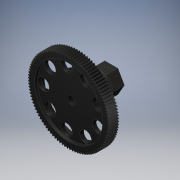
# Autodesk Inventor part: RoueDentée
Saved by Autodesk Inventor 2019 (Build 230136000, 136)
## iProperties
Created: 2019-07-30
Part Number: RoueDentée
Material: Plastique ABS
Document SubType Name: Modeling
Designer: Sébastien DI MERCURIO
Mass: 7.34284 g
Surface Area: 34.3062 cm^2
Volume: 6.92721 cm^3
Density: 1.06 g/cm^3
Appearance: Lustré - Noir
Author: Sébastien DI MERCURIO
Autodesk Inventor part; units mm, degrees
ref_plane "YZ Plane" through (0, 0, 0) normal (1, 0, 0) x (0, 1, 0)
ref_plane "XZ Plane" through (0, 0, 0) normal (0, 1, 0) x (-1, 0, 0)
ref_plane "XY Plane" through (0, 0, 0) normal (0, 0, 1) x (1, 0, 0)
sketch "Esquisse1" plane through (0, 0, 0) normal (0, 0, 1) x (1, 0, 0)
  circle A0 centre (0, 0) radius 21
  dimension "d0" = 42
  constraints: 1 centre point, 1 coincident
  measures "d0" diameter of A0
extrude "Extrusion1" add sketch "Esquisse1" along normal blind 5
sketch "Esquisse2" plane through (0, 0, 5) normal (0, 0, 1) x (1, 0, 0)
  circle A0 centre (0, 0) radius 17.5
  circle A1 centre (0, 0) radius 21 projected
  dimension "d3" = 3.5
  constraints: 1 centre point, 1 coincident
  measures "d3" radial gap between concentric circles of A0 A1
extrude "Extrusion2" cut sketch "Esquisse2" against normal blind 1.5 contours A0
sketch "Esquisse3" plane through (0, 0, 0) normal (0, 0, -1) x (-1, 0, 0)
  circle A0 centre (0, 0) radius 17.5
  circle A1 centre (0, 0) radius 21 projected
  dimension "d6" = 3.5
  constraints: 1 centre point, 1 coincident
  measures "d6" radial gap between concentric circles of A0 A1
extrude "Extrusion3" cut sketch "Esquisse3" against normal blind 1.5 contours A0
sketch "Esquisse4" plane through (0, 0, 1.5) normal (0, 0, -1) x (-1, 0, 0)
  circle A0 centre (0, 0) radius 14.5 construction
  circle A1 centre (14.5, 0) radius 3
  circle A2 centre (11.1076, 9.3204) radius 3
  circle A3 centre (2.5179, 14.2797) radius 3
  circle A4 centre (-7.25, 12.5574) radius 3
  circle A5 centre (-13.6255, 4.9593) radius 3
  circle A6 centre (-13.6255, -4.9593) radius 3
  circle A7 centre (-7.25, -12.5574) radius 3
  circle A8 centre (2.5179, -14.2797) radius 3
  circle A9 centre (11.1076, -9.3204) radius 3
  dimension "d9" = 29
  dimension "d10" = 6
  dimension "d13" = 360
  constraints: 9 centre point, 2 horizontal alignment, 1 coincident, 21 other
  measures "d10" diameter of A1
extrude "Extrusion4" cut sketch "Esquisse4" against normal through all
sketch "Esquisse5" plane through (0, 0, 1.5) normal (0, 0, -1) x (-1, 0, 0)
  circle A0 centre (0, 0) radius 11
  dimension "d17" = 22
  constraints: 1 centre point, 1 coincident
  measures "d17" diameter of A0
extrude "Extrusion5" add sketch "Esquisse5" along normal blind 3
sketch "Esquisse6" plane through (0, 0, -1.5) normal (0, 0, -1) x (-1, 0, 0)
  circle A0 centre (0, 0) radius 6.75
  dimension "d20" = 13.5
  constraints: 1 centre point, 1 coincident
  measures "d20" diameter of A0
extrude "Extrusion6" add sketch "Esquisse6" along normal blind 9.5
sketch "Esquisse9" plane through (0, 0, -11) normal (0, 0, -1) x (-1, 0, 0)
  line L0 (6.75, 0) -> (3.375, -5.8457)
  line L1 (3.375, -5.8457) -> (-3.375, -5.8457)
  line L2 (-3.375, -5.8457) -> (-6.75, 0)
  line L3 (-6.75, 0) -> (-3.375, 5.8457)
  line L4 (-3.375, 5.8457) -> (3.375, 5.8457)
  line L5 (3.375, 5.8457) -> (6.75, 0)
  point P0 (0, 0)
  point P1 (0, 0)
  dimension "d26" = 6.75
  constraints: 12 end point, 2 horizontal alignment, 1 coincident, 13 other
  measures "d26" distance of point (0, 0) L0.start
extrude "Extrusion8" add sketch "Esquisse9" along normal blind 6
sketch "Esquisse7" plane through (0, 0, -11) normal (0, 0, -1) x (-1, 0, 0)
  circle A0 centre (0, 0) radius 2
  dimension "d23" = 4
  constraints: 1 centre point, 1 coincident
  measures "d23" diameter of A0
extrude "Extrusion7" cut sketch "Esquisse7" along normal through all both and the other way through all
sketch "Esquisse10" plane through (0, 0, 5) normal (0, 0, 1) x (1, 0, 0)
  circle A0 centre (0, 0) radius 20 construction
  line L0 (-20, 0) -> (-21.1602, 0.7698)
  line L1 (-21.1602, 0.7698) -> (-21.1602, -0.7698)
  line L2 (-21.1602, -0.7698) -> (-20, 0)
  dimension "d29" = 40
  dimension "d33" = 1.5395
  dimension "d34" = 1.1602
  dimension "d35" = 0.7698
  constraints: 6 end point, 1 coincident, 1 horizontal alignment, 1 vertical, 2 other
  measures "d33" distance of L0.end L1.end
  measures "d34" distance from line of L0.start L1
  measures "d35" vertical distance of point (0, 0) L1.end
extrude "Extrusion9" cut sketch "Esquisse10" against normal through all
pattern_circular "Réseau circulaire1" count 100 over 360 about axis through (0, 0, -11) along (0, 0, -1) of "Extrusion9"
equation "\"d35\" = 0.5 * d33"
